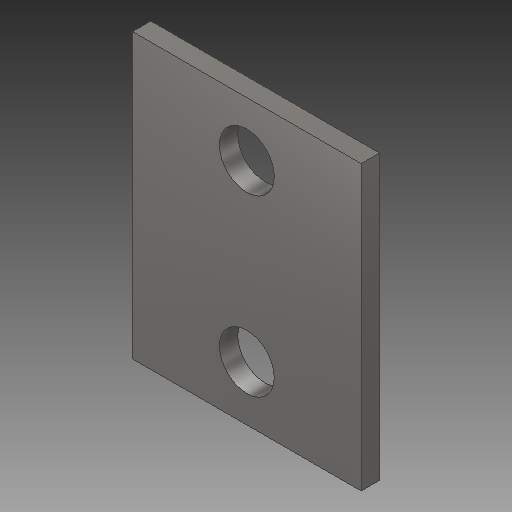
# Autodesk Inventor part: lc_spacer
Saved by Autodesk Inventor 2018.1 (Build 221171000, 171)
## iProperties
Created: 2017-07-29
Part Number: lc_spacer
Material: Stainless Steel
Document SubType Name: Modeling
Designer: Tom
Density: 8 g/cm^3
Appearance: Semi-Polished
Author: Tom
Autodesk Inventor part; units mm, degrees
ref_plane "YZ Plane" through (0, 0, 0) normal (1, 0, 0) x (0, 1, 0)
ref_plane "XZ Plane" through (0, 0, 0) normal (0, 1, 0) x (-1, 0, 0)
ref_plane "XY Plane" through (0, 0, 0) normal (0, 0, 1) x (1, 0, 0)
sketch "Sketch1" plane through (0, 0, 0) normal (0, 0, 1) x (1, 0, 0)
  line L0 (0, 0) -> (25, 0)
  line L1 (25, 0) -> (25, 31)
  line L2 (25, 31) -> (0, 31)
  line L3 (0, 31) -> (0, 0)
  line L4 (12.5, 31) -> (12.5, 0) construction
  line L5 (0, 15.5) -> (25, 15.5) construction
  circle A0 centre (12.5, 25.025) radius 3
  circle A1 centre (12.5, 5.975) radius 3
  dimension "d0" = 25
  dimension "d1" = 31
  dimension "d2" = 6
  dimension "d3" = 19.05
  constraints: 12 end point, 4 midpoint, 2 centre point, 2 parallel, 2 perpendicular, 1 horizontal, 1 point on line, 1 symmetric about line, 2 other
  measures "d0" distance of L2.end L1.end
  measures "d1" distance of L1.end L0.end
  measures "d2" diameter of A0
  measures "d3" diameter of A0.centre L5
extrude "Extrusion1" add sketch "Sketch1" along normal blind 2
equation "\"d0\" = sw"
equation "\"d1\" = sh"
equation "\"d2\" = dia1"
equation "\"d3\" = lcsd"
equation "\"d4\" = spacert"
equation "\"lcsd\" = 19.05"
equation "\"lcwd1\" = 25"
equation "\"lcwd2\" = 34"
equation "\"lch1\" = 39"
equation "\"lcwd3\" = 43"
equation "\"dia1\" = 6"
equation "\"td\" = 18"
equation "\"bhh\" = 6"
equation "\"sw\" = 25"
equation "\"sh\" = 31"
equation "\"spacert\" = 2"
equation "\"pvct\" = 5"
equation "\"dia3\" = 8"
equation "\"dia4\" = 11"
equation "\"tankl\" = 379"
equation "\"play\" = 9"
equation "\"holeh\" = 26"
equation "\"surroundt\" = 5"
equation "\"slack\" = 0.5"
equation "\"play2\" = 3"
equation "\"diaoverflow\" = 25"
equation "\"diawater\" = 25"
equation "\"diacucl\" = 32"
equation "\"diaph\" = 32"
equation "\"diaair\" = 32"
equation "\"diasurroundhole\" = 42"
equation "\"diagrate\" = 12"
equation "\"gratespacing\" = 12.02082"
equation "\"bottomdist\" = 9.6355"
equation "\"sidedist\" = 13.9375"
equation "\"diahcl\" = 32"
equation "\"bracketwtop\" = 6"
equation "\"bracketwbottom\" = 6"
equation "\"nett\" = 1"
equation "\"nethole\" = 16"
equation "\"netside\" = 3.5"
equation "\"nettop\" = 7"
equation "\"netholespacing\" = 2"
equation "\"diaetape\" = 32"
body "Solid1"
